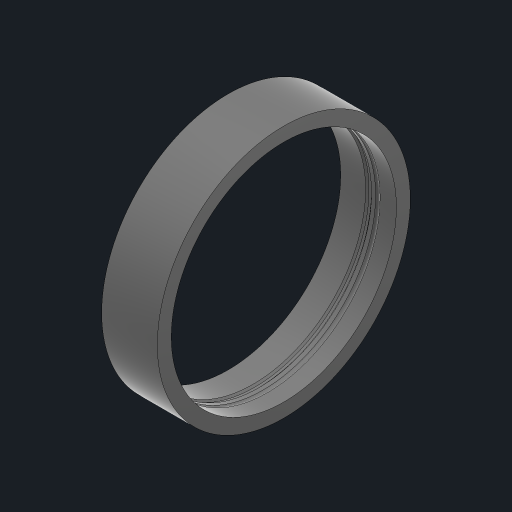
# Autodesk Inventor part: One Piece Ring
Saved by Autodesk Inventor 2023.2 (Build 272271030, 271C)
## iProperties
Created: 2024-02-20
Part Number: One Piece Ring
Material: UHMW, Black
Document SubType Name: Modeling
Designer: robpl
Density: 0.94 g/cm^3
Appearance: Smooth - Black
Mass: 112.614 g
Surface Area: 372.136 cm^2
Volume: 119.802 cm^3
Author: robpl
Autodesk Inventor part; units mm, degrees
ref_plane "YZ Plane" through (0, 0, 0) normal (1, 0, 0) x (0, 1, 0)
ref_plane "XZ Plane" through (0, 0, 0) normal (0, 1, 0) x (-1, 0, 0)
ref_plane "XY Plane" through (0, 0, 0) normal (0, 0, 1) x (1, 0, 0)
sketch "Sketch1" plane through (0, 0, 0) normal (0, 0, 1) x (1, 0, 0)
  line L0 (0, 75) -> (33, 75)
  line L1 (33, 75) -> (33, 66.75)
  line L2 (33, 66.75) -> (0, 66.75)
  line L3 (0, 66.75) -> (0, 75)
  line L4 (14.75, 66.75) -> (15.75, 67.75)
  line L5 (15.75, 67.75) -> (17.25, 67.75)
  line L6 (17.25, 67.75) -> (18.25, 66.75)
  line L7 (15.25, 67.25) -> (17.75, 67.25)
  line L8 (17.75, 67.25) -> (17.75, 66.75)
  line L9 (17.75, 66.75) -> (15.25, 66.75)
  line L10 (15.25, 66.75) -> (15.25, 67.25)
  circle A0 centre (22, 65.25) radius 2
  line L11 (0, -15) -> (0, 90) projected
  line L12 (-6.6, 0) -> (39.6, 0) projected
  point P0 (0, 0)
  point P1 (20, 65.25)
  point P2 (16.5, 67.75)
  point P3 (16.5, 66.75)
  point P4 (20.6771, 66.75)
  point P5 (23.3229, 66.75)
  dimension "d7" = 4
  dimension "d0" = 2.5
  dimension "d1" = 67.25
  dimension "d2" = 0.5
  dimension "d3" = 75
  dimension "d4" = 1
  dimension "d5" = 33
  dimension "d8" = 1.75
  constraints: 22 end point, 4 horizontal, 4 midpoint, 4 parallel, 4 perpendicular, 3 point on line, 2 vertical alignment, 1 horizontal alignment, 3 other
  measures "d0" distance of L7.start L7.end
  measures "d1" distance from line of point (0, 0) L7
  measures "d2" distance between parallel lines of L2 L7
  measures "d3" distance from line of point (0, 0) L0
  measures "d4" distance between parallel lines of L2 L5
  measures "d5" distance of L1.end L2.end
  measures "d8" horizontal distance of L6.end point (20, 65.25)
revolve "Revolution1" add sketch "Sketch1" angle 360 about axis through (-10, 0, 0) along (1, 0, 0) contours L0 L1 L2 A0 L6 L5 L4 L3
body "Solid1"
